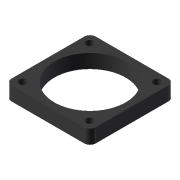
# Autodesk Inventor part: 100_Adapter_Waveplate
Saved by Autodesk Inventor 2019 (Build 230136000, 136)
## iProperties
Created: 2019-07-11
Part Number: 100_Adapter_Waveplate
Material: Generic
Document SubType Name: Modeling
Designer: diederichbenedict
Density: 1 g/cm^3
Appearance: Default
Author: diederichbenedict
Autodesk Inventor part; units mm, degrees
ref_plane "YZ Plane" through (0, 0, 0) normal (1, 0, 0) x (0, 1, 0)
ref_plane "XZ Plane" through (0, 0, 0) normal (0, 1, 0) x (-1, 0, 0)
ref_plane "XY Plane" through (0, 0, 0) normal (0, 0, 1) x (1, 0, 0)
sketch "Sketch1" plane through (0, 0, 0) normal (0, 1, 0) x (-1, 0, 0)
  circle A0 centre (0, 0) radius 12.75
  line L0 (13, 15) -> (-13, 15)
  line L1 (-15, 13) -> (-15, -13)
  line L2 (-13, -15) -> (13, -15)
  line L3 (15, -13) -> (15, 13)
  line L4 (15, 15) -> (-15, -15) construction
  line L5 (-15, 15) -> (15, -15) construction
  arc A1 (15, 13) -> (13, 15) centre (13, 13) ccw
  arc A2 (13, -15) -> (15, -13) centre (13, -13) ccw
  arc A3 (-15, -13) -> (-13, -15) centre (-13, -13) ccw
  arc A4 (-13, 15) -> (-15, 13) centre (-13, 13) ccw
  dimension "d0" = 25.5
  dimension "d1" = 30
  dimension "d2" = 30
  dimension "d3" = 2
  constraints: 12 end point, 8 point on circle, 8 point on line, 8 tangent, 5 centre point, 3 equal radius, 2 midpoint, 2 parallel, 1 coincident, 1 horizontal, 1 perpendicular
  measures "d0" diameter of A0
  measures "d1" distance of L5.end L4.end
  measures "d2" distance of L4.end L5.start
  measures "d3" radius of A1
extrude "Extrusion1" add sketch "Sketch1" along normal blind 5
sketch "Sketch2" plane through (0, 5, 0) normal (0, 1, 0) x (1, 0, 0)
  circle A0 centre (0, 0) radius 12.75 projected
  line L0 (-13, -15) -> (13, -15) projected
  arc A1 (13, -15) -> (15, -13) centre (13, -13) ccw projected
  line L1 (15, -13) -> (15, 13) projected
  arc A2 (15, 13) -> (13, 15) centre (13, 13) ccw projected
  line L2 (13, 15) -> (-13, 15) projected
  arc A3 (-13, 15) -> (-15, 13) centre (-13, 13) ccw projected
  line L3 (-15, 13) -> (-15, -13) projected
  arc A4 (-15, -13) -> (-13, -15) centre (-13, -13) ccw projected
  line L4 (12, 12) -> (-12, 12)
  line L5 (-12, 12) -> (-12, -12)
  line L6 (-12, -12) -> (12, -12)
  line L7 (12, -12) -> (12, 12)
  line L8 (12, 12) -> (-12, -12) construction
  line L9 (-12, 12) -> (12, -12) construction
  dimension "d6" = 24
  dimension "d7" = 24
  dimension "d15" = 30
  constraints: 12 end point, 2 midpoint, 2 parallel, 1 horizontal, 1 perpendicular
  measures "d6" distance of L6.end L5.end
  measures "d7" distance of L5.end L4.end
  measures "d15" distance between parallel lines of L0 L2
hole "Hole1" at (-12, 5, -12) at (12, 5, -12) at (12, 5, 12) at (-12, 5, 12) direction (0, -1, 0) diameter 2.9 depth 24 tip angle 118
body "Solid1"
